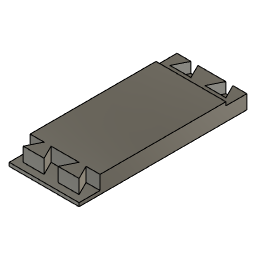
Middle Sword Peice v1 (Autodesk Fusion 360 design; units mm, degrees)
Autodesk Fusion 360 part; units mm, degrees
sketch "Sketch1" plane through (0, 0, 0) normal (0, 1, 0) x (1, 0, 0)
  line L0 (0, 0) -> (100, 0)
  line L1 (100, 0) -> (100, -50)
  line L2 (100, -50) -> (0, -50)
  line L3 (0, -50) -> (0, 0)
  constraint horizontal L0
  constraint vertical L1
  constraint horizontal L2
  constraint vertical L3
  constraint coincident L0.start L3.end
extrude "Extrude1" add sketch "Sketch1" along normal blind 120 makes body 1
extrude "Extrude2" add 1 faces at (33.3333, 120, 16.6667) along direction (0, 1, 0) blind 120 on bodies 1 bodies 1
extrude "Extrude3" cut 1 faces at (66.6667, 80, 50) along direction (0, 0, -1) blind 20 on bodies 1 bodies 1
sketch "Sketch2" plane through (0, 0, 30) normal (0, 0, 1) x (-1, 0, 0)
  line L0 (0, 0) -> (-100, 0)
  line L1 (-100, 0) -> (-100, -240)
  line L2 (-100, -240) -> (0, -240)
  line L3 (0, -240) -> (0, 0)
  line L4 (0, -30) -> (-20, -30)
  line L5 (-20, -30) -> (-10, -10)
  line L6 (-10, -10) -> (-40, -10)
  line L7 (-40, -10) -> (-30, -30)
  line L8 (-30, -30) -> (-50, -30)
  line L9 (-50, -30) -> (-70, -30)
  line L10 (-70, -30) -> (-60, -10)
  line L11 (-60, -10) -> (-90, -10)
  line L12 (-90, -10) -> (-80, -30)
  line L13 (-80, -30) -> (-100, -30)
  line L14 (-100, -240) -> (0, -240)
  constraint coincident L3 L4.start
  constraint perpendicular L3 L4
  constraint perpendicular L3 L6
  constraint parallel L6 L8
  constraint parallel L8 L9
  constraint parallel L9 L11
  constraint coincident L1 L13.end
  constraint perpendicular L1 L13
  constraint coincident L1.end L2.start
  constraint coincident L2.end L3.start
extrude "Extrude4" add sketch "Sketch2" along normal blind 20 contours L1 L2 L3 L4 L5 L6 L7 L8 L9 L10 L11 L12 L13 L14 bodies 1
extrude "Extrude5" cut 1 faces at (33.3333, 80, 0) along direction (0, 0, 1) blind 25 on bodies 1 bodies 1
pattern_linear "R-Pattern1" count 2 spacing 250 along (1, 0, 0) of bodies 1 makes body 2
move_body "Move1" bodies 2 to x (1, 0, 0) y (0, 1, 0) z (0, 0, 1) at (-110, 0, 0)
move_body "Move4" bodies 1 to x (1, 0, 0) y (0, 1, 0) z (0, 0, 1) at (140, 210, 10)
move_body "Move5" bodies 1 to x (1, 0, 0) y (0, 1, 0) z (0, 0, 1) at (0, 40, 0)
sketch "Sketch7" plane through (0, 0, 50) normal (0, 0, 1) x (-1, 0, 0)
  line L0 (-240, -240) -> (-140, -240)
  line L1 (-140, -240) -> (-140, -30)
  line L2 (-140, -30) -> (-160, -30)
  line L3 (-160, -30) -> (-150, -10)
  line L4 (-150, -10) -> (-180, -10)
  line L5 (-180, -10) -> (-170, -30)
  line L6 (-170, -30) -> (-210, -30)
  line L7 (-210, -30) -> (-200, -10)
  line L8 (-200, -10) -> (-230, -10)
  line L9 (-230, -10) -> (-220, -30)
  line L10 (-220, -30) -> (-240, -30)
  line L11 (-240, -30) -> (-240, -240)
  line L12 (-240, -210) -> (-140, -210)
  line L13 (-140, -240) -> (-160, -240)
  line L14 (-150, -220) -> (-180, -220)
  line L15 (-180, -220) -> (-170, -240)
  line L16 (-210, -240) -> (-200, -220)
  line L17 (-200, -220) -> (-230, -220)
  line L18 (-230, -220) -> (-220, -240)
  line L19 (-240, -240) -> (-240, -210)
  line L20 (-150, -220) -> (-160, -240)
  constraint coincident L11 L12.start
  constraint coincident L1 L12.end
  constraint perpendicular L1 L12
  constraint coincident L0.end L1.start
  constraint coincident L0 L13.end
  constraint perpendicular L1 L13
  constraint perpendicular L1 L14
  constraint coincident L0 L15.end
  constraint coincident L0 L16.start
  constraint parallel L0 L17
  constraint coincident L0 L18.end
  constraint parallel L15 L18
  constraint coincident L0.start L11.end
move_body "Move6" bodies 1 to x (1, 0, 0) y (0, 1, 0) z (0, 0, 1) at (140, 0, 0)
extrude "Extrude6" cut sketch "Sketch7" against normal blind 20 contours L0 L16 L17 L18 | L0 L14 L15 L20 bodies 2
sketch "Sketch8" plane through (0, 0, 50) normal (0, 0, 1) x (-1, 0, 0)
  line L0 (-220, -240) -> (-230, -220)
  line L1 (-230, -220) -> (-200, -220)
  line L2 (-200, -220) -> (-210, -240)
  line L3 (-210, -240) -> (-170, -240)
  line L4 (-170, -240) -> (-180, -220)
  line L5 (-180, -220) -> (-150, -220)
  line L6 (-150, -220) -> (-160, -240)
  line L7 (-160, -240) -> (-140, -240)
  line L8 (-140, -240) -> (-140, -30)
  line L9 (-140, -30) -> (-160, -30)
  line L10 (-160, -30) -> (-150, -10)
  line L11 (-150, -10) -> (-180, -10)
  line L12 (-180, -10) -> (-170, -30)
  line L13 (-170, -30) -> (-210, -30)
  line L14 (-210, -30) -> (-200, -10)
  line L15 (-200, -10) -> (-230, -10)
  line L16 (-230, -10) -> (-220, -30)
  line L17 (-220, -30) -> (-240, -30)
  line L18 (-240, -30) -> (-240, -240)
  line L19 (-240, -240) -> (-220, -240)
  line L20 (-240, -210) -> (-140, -210)
  line L21 (-140, -240) -> (-160, -240)
  line L22 (-150, -220) -> (-180, -220)
  line L23 (-170, -240) -> (-210, -240)
  line L24 (-200, -220) -> (-230, -220)
  line L25 (-220, -240) -> (-240, -240)
  constraint coincident L18 L20.start
  constraint coincident L8 L20.end
  constraint perpendicular L8 L20
  constraint coincident L7.end L8.start
  constraint coincident L6.end L7.start
  constraint coincident L5.end L6.start
  constraint coincident L4.end L5.start
  constraint coincident L3.end L4.start
  constraint coincident L2.end L3.start
  constraint coincident L1.end L2.start
  constraint coincident L0.end L1.start
  constraint coincident L0.start L19.end
  constraint coincident L18.end L19.start
extrude "Extrude7" cut sketch "Sketch8" against normal blind 5 contours L0 L1 L2 L3 L4 L5 L6 L7 L8 L18 L19 L20 L21 L22 L23 L24 L25 bodies 2
move_body "Move7" bodies 1 to x (-1, 0, 0) y (0, 1, 0) z (0, 0, -1) at (514.0176, -40, 85)
move_body "Move8" bodies 1 to x (1, 0, 0) y (0, 1, 0) z (0, 0, 1) at (5, 0, 0)
move_body "Move9" bodies 1 to x (1, 0, 0) y (0, 1, 0) z (0, 0, 1) at (-190, 0, 0)
copy_body "CopyPasteBodies1" bodies 2 makes body 3
move_body "Move10" bodies 3 to x (-1, 0, 0) y (0, 1, 0) z (0, 0, -1) at (381.7693, 210, 75)
move_body "Move11" bodies 3 to x (1, 0, 0) y (0, 1, 0) z (0, 0, 1) at (-2, 0, 0)
move_body "Move12" bodies 3 to x (1, 0, 0) y (0, 1, 0) z (0, 0, 1) at (0.23, 0, 0)
move_body "Move13" bodies 2 to x (1, 0, 0) y (0, -1, 0) z (0, 0, -1) at (0, 71.5148, 26.5138)
move_body "Move14" bodies 2 to x (1, 0, 0) y (0, 1, 0) z (0, 0, 1) at (0, 168.4192, -1.355)
move_body "Move15" bodies 2 to x (1, 0, 0) y (0, 1, 0) z (0, 0, 1) at (0, -230, 25)
move_body "Move16" bodies 2 to x (1, 0, 0) y (0, 1, 0) z (0, 0, 1) at (0, -10, 0)
move_body "Move17" bodies 2 to x (1, 0, 0) y (0, -1, 0) z (0, 0, -1) at (0, -0.1319, 25.3178)
move_body "Move18" bodies 2 to x (1, 0, 0) y (0, 1, 0) z (0, 0, 1) at (-140, 0, 0)
hidden bodies 1 3
